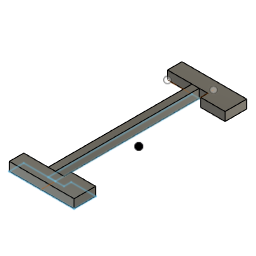
Wheel Arm Base v1 (Autodesk Fusion 360 design; units mm, degrees)
Autodesk Fusion 360 part; units mm, degrees
note: some values were not read from the file. Set by a fixed rule: which sketch regions a step uses.
sketch "Sketch1" plane through (0, 0, 0) normal (0, 0, 1) x (1, 0, 0)
  line L0 (-30, 50) -> (-8, 50) construction
  line L1 (-8, 50) -> (-8, 60) construction
  line L2 (-8, 50) -> (-8, -60) construction
  line L3 (-8, -60) -> (-8, -50) construction
  line L4 (-8, -50) -> (-2, -50)
  line L5 (-2, -50) -> (-2, -45)
  line L6 (-2, -45) -> (15, -45)
  line L7 (15, -45) -> (15, -60)
  line L8 (-8, -50) -> (-30, -50)
  line L9 (-30, -50) -> (-30, -60)
  line L10 (-30, -60) -> (15, -60)
  line L11 (-8, 50) -> (-13, 50)
  line L12 (-13, 50) -> (-13, -50)
  line L13 (-13, -50) -> (-8, -50)
  line L14 (-8, -50) -> (-8, 50)
  dimension "d3" = 22
  dimension "d4" = 17
  dimension "d10" = 5
  constraint coincident L2 L3.end
  constraint perpendicular L2 L4
  constraint perpendicular L4 L5
  constraint perpendicular L2 L6
  constraint horizontal L11
  constraint vertical L12
  constraint horizontal L13
  constraint vertical L14
  constraint coincident L8 L12.end
  measures "d3" distance of L0.start L0.end
  measures "d4" distance of L5.end L6.end
  measures "d10" distance of L0.end L11.end
extrude "Extrude1" add sketch "Sketch1" along normal blind 6 contours L4 L5 L6 L7 L8 L9 L10 L13 makes body 1
ref_plane "WorkPlane1" through (0, 0, 0) normal (0, 1, 0) x (0, 0, 1)
mirror "Mirror1" about plane through (0, 0, 0) normal (0, 1, 0) of bodies 1 makes body 2
extrude "Extrude2" add sketch "Sketch1" along normal blind 6 separate body contours L8 L11 L12 L13 L14 makes body 3
